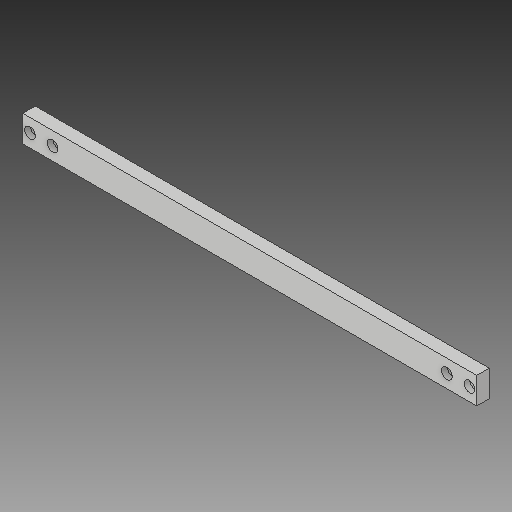
# Autodesk Inventor part: suporte_esbarro_barro
Saved by Autodesk Inventor 2018 (Build 220112000, 112)
## iProperties
Created: 2018-05-17
Part Number: suporte_esbarro_barro
Material: Genérico
Document SubType Name: Modeling
Designer: Usuario
Density: 1 g/cm^3
Appearance: Padrão
Author: Usuario
Autodesk Inventor part; units mm, degrees
ref_plane "YZ Plane" through (0, 0, 0) normal (1, 0, 0) x (0, 1, 0)
ref_plane "XZ Plane" through (0, 0, 0) normal (0, 1, 0) x (-1, 0, 0)
ref_plane "XY Plane" through (0, 0, 0) normal (0, 0, 1) x (1, 0, 0)
sketch "Esboço1" plane through (0, 0, 0) normal (0, 0, 1) x (1, 0, 0)
  circle A0 centre (5.5, 10) radius 1.621 construction
  circle A1 centre (22.5, 10) radius 1.621 construction
  line L0 (28, 0) -> (0, 0) construction
  line L1 (28, 0) -> (28, 20) construction
  line L2 (0, 20) -> (28, 20) construction
  line L3 (0, 0) -> (0, 20) construction
  circle A2 centre (-309.5, 10) radius 1.621 construction
  circle A3 centre (-292.5, 10) radius 1.621 construction
  line L4 (-287, 0) -> (-315, 0) construction
  line L5 (-287, 0) -> (-287, 20) construction
  line L6 (-315, 20) -> (-287, 20) construction
  line L7 (-315, 0) -> (-315, 20) construction
  line L8 (28, 0) -> (-315, 0)
  line L9 (-315, 0) -> (-315, 20)
  line L10 (-315, 20) -> (28, 20)
  line L11 (28, 20) -> (28, 0)
  circle A4 centre (22.5, 10) radius 1.621 construction
  circle A5 centre (5.5, 10) radius 1.621 construction
  circle A6 centre (-292.5, 10) radius 1.621 construction
  circle A7 centre (-309.5, 10) radius 1.621 construction
  constraints: 8 end point, 4 centre point, 4 coincident, 4 concentric, 2 parallel, 1 horizontal, 1 perpendicular
extrude "Extrusão1" add sketch "Esboço1" along normal blind 9.5
sketch "Esboço3" plane through (0, 0, 9.5) normal (0, 0, 1) x (1, 0, 0)
  circle A0 centre (22.5, 10) radius 1.621 construction
  circle A1 centre (5.5, 10) radius 1.621 construction
  circle A2 centre (-292.5, 10) radius 1.621 construction
  circle A3 centre (-309.5, 10) radius 1.621 construction
  point P0 (0, 0)
hole "Furo2" at (22.5, 10, 9.5) at (5.5, 10, 9.5) at (-309.5, 10, 9.5) at (-292.5, 10, 9.5) direction (0, 0, -1) diameter 4 end through all counterbore diameter 8 counterbore depth 4.3
